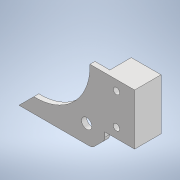
# Autodesk Inventor part: Y-LIMIT SWITCH PLATE
Saved by Autodesk Inventor 2020 (Build 240168000, 168)
## iProperties
Created: 2019-10-11
Part Number: Y-LIMIT SWITCH PLATE
Material: Generic
Document SubType Name: Modeling
Designer: pepd9
Density: 1 g/cm^3
Appearance: Default
Author: pepd9
Autodesk Inventor part; units mm, degrees
ref_plane "YZ Plane" through (0, 0, 0) normal (1, 0, 0) x (0, 1, 0)
ref_plane "XZ Plane" through (0, 0, 0) normal (0, 1, 0) x (-1, 0, 0)
ref_plane "XY Plane" through (0, 0, 0) normal (0, 0, 1) x (1, 0, 0)
sketch "Sketch1" plane through (0, 0, 0) normal (0, 0, 1) x (1, 0, 0)
  line L0 (20.0607, 17.4322) -> (17.4322, 20.0607)
  arc A0 (17.4322, 20.0607) -> (16.3716, 20.5) centre (16.3716, 19) ccw
  line L1 (16.3716, 20.5) -> (-16.3716, 20.5)
  arc A1 (-16.3716, 20.5) -> (-17.4322, 20.0607) centre (-16.3716, 19) ccw
  line L2 (-17.4322, 20.0607) -> (-20.0607, 17.4322)
  arc A2 (-20.0607, 17.4322) -> (-20.5, 16.3716) centre (-19, 16.3716) ccw
  line L3 (-20.5, 16.3716) -> (-20.5, -16.3716)
  arc A3 (-20.5, -16.3716) -> (-20.0607, -17.4322) centre (-19, -16.3716) ccw
  line L4 (-20.0607, -17.4322) -> (-17.4322, -20.0607)
  arc A4 (-17.4322, -20.0607) -> (-16.3716, -20.5) centre (-16.3716, -19) ccw
  line L5 (-16.3716, -20.5) -> (16.3716, -20.5)
  arc A5 (16.3716, -20.5) -> (17.4322, -20.0607) centre (16.3716, -19) ccw
  line L6 (17.4322, -20.0607) -> (20.0607, -17.4322)
  arc A6 (20.0607, -17.4322) -> (20.5, -16.3716) centre (19, -16.3716) ccw
  line L7 (20.5, -16.3716) -> (20.5, 16.3716)
  arc A7 (20.5, 16.3716) -> (20.0607, 17.4322) centre (19, 16.3716) ccw
  circle A8 centre (0, 0) radius 16.5
  circle A9 centre (15.5, 15.5) radius 1.55
  circle A10 centre (15.5, -15.5) radius 1.55
  circle A11 centre (-15.5, -15.5) radius 1.55
  circle A12 centre (-15.5, 15.5) radius 1.55
  line L8 (0, -13) -> (0, -16)
  line L9 (0, -13) -> (-1.914, -11.086)
  arc A13 (-11.25, 0) -> (-1.914, -11.086) centre (0, 0) ccw
  line L10 (-11.25, 0) -> (-11.25, -10.75)
  line L11 (-11.25, -10.75) -> (-21, -10.75)
  line L12 (-21, -10.75) -> (-21, -21)
  line L13 (-21, -21) -> (-5, -21)
  line L14 (-5, -21) -> (0, -16)
  circle A14 centre (-15.5, -15.5) radius 2.8
  line L15 (20.5, -5.5) -> (15.5563, -5.5)
  line L16 (21, 16.3716) -> (21, -16.3716)
  line L17 (21, -16.3716) -> (20.5, -16.3716)
  arc A15 (20.4142, -17.7858) -> (21, -16.3716) centre (19, -16.3716) ccw
  line L18 (20.4142, -17.7858) -> (17.7858, -20.4142)
  arc A16 (16.3716, -21) -> (17.7858, -20.4142) centre (16.3716, -19) ccw
  line L19 (16.3716, -21) -> (-16.3716, -21)
  line L20 (20.5, -5.5) -> (21, -5.5)
  point P0 (0, 0)
  point P1 (-0.4926, -16.4926)
  point P2 (-4.5, -20.5)
extrude "Extrusion1" add sketch "Sketch1" along normal blind 1.5 contours L20 L16 L17 L7 | L7 A6 L6 A5 L5 L14 A8 L15 | L17 A15 L18 A16 L19 L14 L5 A5 L6 A6
sketch "Sketch2" plane through (0, 0, 1.5) normal (0, 0, 1) x (1, 0, 0)
  circle A0 centre (24.5, -12) radius 0.95
  circle A1 centre (24.5, -2.5) radius 0.95
  line L0 (30, 0.5) -> (21, 0.5)
  line L1 (21, 0.5) -> (21, -15)
  line L2 (21, -15) -> (30, -15)
  line L3 (30, -15) -> (30, 0.5)
  point P0 (0, 0)
  point P1 (21, -5.5)
  dimension "d4" = 24.5
  dimension "d5" = 24.5
  dimension "d6" = 9.5
  dimension "d7" = 1.9
  dimension "d8" = 1.9
  dimension "d9" = 12
  dimension "d10" = 3
  dimension "d11" = 9
  dimension "d12" = 3
  constraints: 8 end point, 2 centre point, 2 parallel, 1 horizontal, 1 perpendicular, 1 point on line
  measures "d4" horizontal distance of point (0, 0) A1.centre
  measures "d5" horizontal distance of point (0, 0) A0.centre
  measures "d6" distance of A0.centre A1.centre
  measures "d7" diameter of A0
  measures "d8" diameter of A1
  measures "d9" vertical distance of point (0, 0) A0.centre
  measures "d10" distance from line of L2 A0.centre
  measures "d11" distance of L1.end L2.end
  measures "d12" distance from line of L0 A1.centre
extrude "Extrusion2" add sketch "Sketch2" against normal blind 8
sketch "Sketch3" plane through (0, 0, 1.5) normal (0, 0, 1) x (1, 0, 0)
  arc A0 (-0.4926, -16.4926) -> (15.5563, -5.5) centre (0, 0) ccw projected
  circle A1 centre (24.5, -2.5) radius 0.95 projected
  circle A2 centre (24.5, -12) radius 0.95 projected
  line L0 (-0.4926, -16.4926) -> (-5, -21) projected
  line L1 (-5, -21) -> (16.3716, -21) projected
  arc A3 (16.3716, -21) -> (17.7858, -20.4142) centre (16.3716, -19) ccw projected
  line L2 (17.7858, -20.4142) -> (20.4142, -17.7858) projected
  arc A4 (20.4142, -17.7858) -> (21, -16.3716) centre (19, -16.3716) ccw projected
  line L3 (21, 0.5) -> (21, -5.5) projected
  line L4 (21, -15) -> (30, -15) projected
  line L5 (30, -15) -> (30, 0.5) projected
  line L6 (30, 0.5) -> (21, 0.5) projected
  line L7 (21, -5.5) -> (15.5563, -5.5) projected
  arc A5 (-0.4926, -16.4926) -> (15.5563, -5.5) centre (0, 0) ccw projected
  circle A6 centre (15.5, -15.5) radius 1.55 projected
  circle A7 centre (0, 0) radius 16.5
  line L8 (21, 0.5) -> (16.4924, 0.5)
  line L9 (21, -15) -> (30, -15) projected
  line L10 (22.3286, -15) -> (17.1369, -20.8478)
  arc A8 (16.3716, -21) -> (17.7858, -20.4142) centre (16.3716, -19) ccw projected
  line L11 (21, -16.3716) -> (21, -15) projected
  point P0 (0, 0)
  point P1 (21, -17)
  point P2 (15.5563, -5.5)
  point P3 (17.2535, -20.795)
  point P4 (17.9687, -20.2313)
  constraints: 4 end point, 4 point on circle, 1 centre point, 1 coincident, 1 horizontal, 2 other
extrude "Extrusion3" add sketch "Sketch3" against normal blind 1.5 contours A7 L8 L3 L7
body "Solid1"
